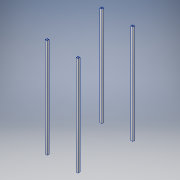
# Autodesk Inventor part: supportForLift
Saved by Autodesk Inventor 2018.2 (Build 222227000, 227)
## iProperties
Created: 2018-01-07
Part Number: supportForLift
Material: Aluminum 6061
Document SubType Name: Modeling
Designer: steele
Density: 2.7 g/cm^3
Appearance: Aluminum - Flat
Mass: 3871.44 g
Surface Area: 9054.82 cm^2
Volume: 1433.87 cm^3
Author: steele
Autodesk Inventor part; units mm, degrees
ref_plane "YZ Plane" through (0, 0, 0) normal (1, 0, 0) x (0, 1, 0)
ref_plane "XZ Plane" through (0, 0, 0) normal (0, 1, 0) x (-1, 0, 0)
ref_plane "XY Plane" through (0, 0, 0) normal (0, 0, 1) x (1, 0, 0)
sketch "Sketch1" plane through (0, 0, 0) normal (0, 1, 0) x (-1, 0, 0)
  line L0 (206.375, 356.362) -> (-206.375, 356.362) construction
  line L1 (-206.375, 356.362) -> (-206.375, -356.362) construction
  line L2 (-206.375, -356.362) -> (206.375, -356.362) construction
  line L3 (206.375, -356.362) -> (206.375, 356.362) construction
  line L4 (206.375, 356.362) -> (-206.375, -356.362) construction
  line L5 (-206.375, 356.362) -> (206.375, -356.362) construction
  line L6 (-206.375, -356.362) -> (-180.975, -356.362)
  line L7 (-180.975, -356.362) -> (-180.975, -330.962)
  line L8 (-180.975, -330.962) -> (-206.375, -330.962)
  line L9 (-206.375, -330.962) -> (-206.375, -356.362)
  line L10 (-203.2, -334.137) -> (-184.15, -334.137)
  line L11 (-184.15, -334.137) -> (-184.15, -353.187)
  line L12 (-184.15, -353.187) -> (-203.2, -353.187)
  line L13 (-203.2, -353.187) -> (-203.2, -334.137)
  line L14 (-203.2, -334.137) -> (-184.15, -353.187) construction
  line L15 (-184.15, -334.137) -> (-203.2, -353.187) construction
  point P0 (0, 0)
  point P1 (-193.675, -343.662)
  dimension "d0" = 412.75
  dimension "d1" = 712.724
  dimension "d2" = 25.4
  dimension "d3" = 25.4
  dimension "d4" = 19.05
  dimension "d5" = 19.05
  constraints: 32 end point, 6 parallel, 4 midpoint, 3 horizontal, 3 perpendicular
  measures "d0" distance of L0.start L0.end
  measures "d1" distance of L1.end L0.end
  measures "d2" distance of L8.end L7.end
  measures "d3" distance of L7.end L6.end
  measures "d4" distance of L10.start L10.end
  measures "d5" distance of L10.end L11.end
extrude "Extrusion1" add sketch "Sketch1" against normal blind 1244.6
mirror "Mirror1" about plane through (0, 0, 0) normal (1, 0, 0) of "Extrusion1"
mirror "Mirror2" about plane through (0, 0, 0) normal (0, 0, 1) of "Extrusion1", "Mirror1"
body "Solid1"
